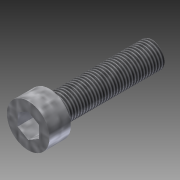
# Autodesk Inventor part: M4
Saved by Autodesk Inventor 2015 (Build 190159000, 159)
## iProperties
Created: 2016-11-27
Part Number: M4
Material: Generic
Document SubType Name: Modeling
Designer: Hampus
Density: 1 g/cm^3
Appearance: Aluminum Cast
Author: Hampus
Autodesk Inventor part; units mm, degrees
ref_plane "YZ Plane" through (0, 0, 0) normal (1, 0, 0) x (0, 1, 0)
ref_plane "XZ Plane" through (0, 0, 0) normal (0, 1, 0) x (-1, 0, 0)
ref_plane "XY Plane" through (0, 0, 0) normal (0, 0, 1) x (1, 0, 0)
sketch "Sketch1" plane through (0, 0, 0) normal (0, 1, 0) x (-1, 0, 0)
  circle A0 centre (0, 0) radius 1.5
  circle A1 centre (0, 0) radius 2.5
  dimension "d0" = 3
  dimension "d1" = 5
  constraints: 2 centre point, 2 coincident
  measures "d0" diameter of A0
  measures "d1" diameter of A1
extrude "Extrusion1" add sketch "Sketch1" along normal blind 12 contours A0
extrude "Extrusion2" add sketch "Sketch1" against normal blind 2.5 contours A0 | A1
thread "Thread1" size "M3x0.35" class "6g" standard "ANSI Metric M Profile" full length
sketch "Sketch2" plane through (0, -2.5, 0) normal (0, -1, 0) x (1, 0, 0)
  line L0 (1.25, -0.7217) -> (0, -1.4434)
  line L1 (0, -1.4434) -> (-1.25, -0.7217)
  line L2 (-1.25, -0.7217) -> (-1.25, 0.7217)
  line L3 (-1.25, 0.7217) -> (0, 1.4434)
  line L4 (0, 1.4434) -> (1.25, 0.7217)
  line L5 (1.25, 0.7217) -> (1.25, -0.7217)
  point P0 (0, 0)
  point P1 (0, 0)
  point P2 (1.25, 0)
  constraints: 12 end point, 1 midpoint, 13 other
extrude "Extrusion3" cut sketch "Sketch2" against normal blind 2
body "Solid1"
